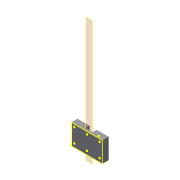
# Autodesk Inventor part: 04_Mount_Rail_Fastener
Saved by Autodesk Inventor 2019.4 (Build 234330000, 330)
## iProperties
Created: 2021-02-16
Part Number: 04_Mount_Rail_Fastener
Material: Generic
Document SubType Name: Modeling
Designer: diederichbenedict
Density: 1 g/cm^3
Appearance: Default
Author: diederichbenedict
Autodesk Inventor part; units mm, degrees
ref_plane "YZ Plane" through (0, 0, 0) normal (1, 0, 0) x (0, 1, 0)
ref_plane "XZ Plane" through (0, 0, 0) normal (0, 1, 0) x (-1, 0, 0)
ref_plane "Work Plane1" through (22.0339, 196.5, 8) normal (0, 0, 1) x (1, 0, 0)
sketch "Sketch1" plane through (22.0339, 196.5, 8) normal (0, 0, 1) x (1, 0, 0)
  circle A0 centre (5.4838, -190) radius 1.4 projected
  circle A1 centre (27.9838, -190) radius 1.4 projected
  circle A2 centre (-17.0162, -190) radius 1.4 projected
  line L0 (-22.0339, -196.5) -> (32.9661, -196.5) projected
  line L1 (32.9661, -196.5) -> (32.9661, -186.5) projected
  line L2 (-22.0339, -186.5) -> (32.9661, -186.5) projected
  line L3 (-22.0339, -196.5) -> (-22.0339, -186.5) projected
  circle A3 centre (27.9838, -165) radius 1.4 projected
  circle A4 centre (-17.0162, -165) radius 1.4 projected
  circle A5 centre (5.4838, -165) radius 1.4 projected
  line L4 (32.9661, -160.5) -> (32.9661, -169.5) projected
  line L5 (-22.0339, -160.5) -> (32.9661, -160.5) projected
  line L6 (-22.0339, -160.5) -> (-22.0339, -169.5) projected
  line L7 (32.9661, -169.5) -> (-22.0339, -169.5) projected
  line L8 (32.9661, -196.5) -> (-22.0339, -196.5)
  line L9 (-22.0339, -196.5) -> (-22.0339, -160.5)
  line L10 (-22.0339, -160.5) -> (32.9661, -160.5)
  line L11 (32.9661, -160.5) -> (32.9661, -196.5)
  constraints: 8 end point, 2 parallel, 1 horizontal, 1 perpendicular
extrude "Extrusion1" add sketch "Sketch1" along normal blind 4
sketch "Sketch2" plane through (22.0339, 196.5, 8) normal (0, 0, -1) x (-1, 0, 0)
  circle A0 centre (17.0162, -190) radius 1.4 projected
  circle A1 centre (-27.9838, -190) radius 1.4 projected
  circle A2 centre (-5.4838, -190) radius 1.4 projected
  circle A3 centre (-5.4838, -165) radius 1.4 projected
  circle A4 centre (17.0162, -165) radius 1.4 projected
  circle A5 centre (-27.9838, -165) radius 1.4 projected
  line L0 (-32.9661, -196.5) -> (-32.9661, -160.5) projected
  line L1 (22.0339, -196.5) -> (-32.9661, -196.5) projected
  line L2 (22.0339, -160.5) -> (22.0339, -196.5) projected
  line L3 (-32.9661, -160.5) -> (22.0339, -160.5) projected
  line L4 (22.0339, -196.5) -> (-32.9661, -196.5) projected
  line L5 (22.0339, -160.5) -> (0.6985, -160.5)
  line L6 (0.6985, -160.5) -> (0.6985, -196.5)
  line L7 (0.6985, -196.5) -> (22.0339, -196.5)
  line L8 (22.0339, -196.5) -> (22.0339, -160.5)
  line L9 (-32.9661, -196.5) -> (-32.9661, -160.5) projected
  line L10 (-32.9661, -160.5) -> (-11.6661, -160.5)
  line L11 (-11.6661, -160.5) -> (-11.6661, -196.5)
  line L12 (-11.6661, -196.5) -> (-32.9661, -196.5)
  line L13 (-32.9661, -196.5) -> (-32.9661, -160.5)
  line L14 (-11.4661, 0) -> (-11.4661, -200) projected
  line L15 (0.4985, 0) -> (0.4985, -200) projected
  dimension "d6" = 0.2
  dimension "d7" = 0.2
  constraints: 16 end point, 4 parallel, 2 horizontal, 2 perpendicular, 2 point on line
  measures "d6" distance between parallel lines of L15 L6
  measures "d7" distance between parallel lines of L14 L11
extrude "Extrusion2" add sketch "Sketch2" along normal blind 7 contours L0 L3 L11 L1 | L6 L3 L2 L1
sketch "Sketch3" plane through (22.0339, 196.5, 12) normal (0, 0, 1) x (1, 0, 0)
  circle A0 centre (-17.0162, -190) radius 1.4 projected
  circle A1 centre (27.9838, -190) radius 1.4 projected
  circle A2 centre (5.4838, -190) radius 1.4 projected
  circle A3 centre (5.4838, -165) radius 1.4 projected
  circle A4 centre (-17.0162, -165) radius 1.4 projected
  circle A5 centre (27.9838, -165) radius 1.4 projected
  line L0 (32.9661, -196.5) -> (32.9661, -160.5) projected
  line L1 (32.9661, -160.5) -> (-22.0339, -160.5) projected
  line L2 (-22.0339, -160.5) -> (-22.0339, -196.5) projected
  line L3 (-22.0339, -196.5) -> (32.9661, -196.5) projected
  circle A6 centre (28.987, -157.2) radius 1 projected
  circle A7 centre (28.987, -157.2) radius 1 projected
  circle A8 centre (50.837, -147.5) radius 1 projected
  line L4 (53.837, -158.2) -> (53.837, -154.2581) projected
  line L5 (53.837, -154.2581) -> (61.5817, -154.2581) projected
  line L6 (61.5817, -154.2581) -> (61.5817, -153.1829) projected
  line L7 (61.5817, -153.1829) -> (53.837, -153.1829) projected
  line L8 (53.837, -153.1829) -> (53.837, -149.448) projected
  line L9 (53.837, -149.448) -> (61.5817, -149.448) projected
  line L10 (61.5817, -149.448) -> (61.5817, -148.769) projected
  line L11 (61.5817, -148.769) -> (53.837, -148.769) projected
  line L12 (53.837, -148.769) -> (53.837, -146.5) projected
  arc A9 (53.837, -146.5) -> (51.837, -144.5) centre (51.837, -146.5) ccw projected
  line L13 (51.837, -144.5) -> (46.3523, -144.5) projected
  line L14 (46.3523, -144.5) -> (18.7709, -139.6366) projected
  line L15 (18.7709, -139.6366) -> (16.0392, -139.155) projected
  line L16 (16.0392, -139.155) -> (15.987, -139.4512) projected
  line L17 (15.987, -139.4512) -> (44.6201, -144.5) projected
  line L18 (44.6201, -144.5) -> (27.987, -144.5) projected
  arc A10 (27.987, -144.5) -> (25.987, -146.5) centre (27.987, -146.5) ccw projected
  line L19 (25.987, -146.5) -> (25.987, -158.2) projected
  arc A11 (25.987, -158.2) -> (27.987, -160.2) centre (27.987, -158.2) ccw projected
  line L20 (27.987, -160.2) -> (33.9661, -160.2) projected
  line L21 (33.9661, -164.2178) -> (33.9661, -160.2) projected
  line L22 (42.5677, -164.2178) -> (33.9661, -164.2178) projected
  line L23 (42.5677, -164.2178) -> (42.5677, -163.1992) projected
  line L24 (42.5677, -163.1992) -> (35.1545, -163.1992) projected
  line L25 (35.1545, -160.2) -> (35.1545, -163.1992) projected
  line L26 (35.1545, -160.2) -> (51.837, -160.2) projected
  arc A12 (51.837, -160.2) -> (53.837, -158.2) centre (51.837, -158.2) ccw projected
  line L27 (32.9661, -160.5) -> (-22.0339, -160.5) projected
  line L28 (20.9661, -160.5) -> (32.9661, -160.5)
  line L29 (32.9661, -160.5) -> (32.9661, -144.5)
  line L30 (32.9661, -144.5) -> (20.9661, -144.5)
  line L31 (20.9661, -144.5) -> (20.9661, -160.5)
  point P0 (-22.0339, -196.5)
  dimension "d8" = 12
  constraints: 8 end point, 3 point on line, 2 parallel, 1 horizontal, 1 perpendicular
  measures "d8" distance between parallel lines of L31 L29
ref_plane "Work Plane2" through (38.0184, 32.2776, 9) normal (0, 0, 1) x (1, 0, 0)
extrude "Extrusion3" add sketch "Sketch3" against normal up to surface (3 mm away) contours L1 L31 L30 A10 L19 A11 L20 L29 | L20 A11 L19 A10 L18 L29
sketch "Sketch4" plane through (55, 52, 9) normal (0, 0, -1) x (-1, 0, 0)
  circle A0 centre (3.9791, -12.7) radius 1 projected
  circle A1 centre (-17.8709, -3) radius 1 projected
  line L0 (-20.8709, -13.7) -> (-20.8709, -9.7581) projected
  line L1 (-20.8709, -9.7581) -> (-28.6156, -9.7581) projected
  line L2 (-28.6156, -9.7581) -> (-28.6156, -8.6829) projected
  line L3 (-28.6156, -8.6829) -> (-20.8709, -8.6829) projected
  line L4 (-20.8709, -8.6829) -> (-20.8709, -4.948) projected
  line L5 (-20.8709, -4.948) -> (-28.6156, -4.948) projected
  line L6 (-28.6156, -4.948) -> (-28.6156, -4.269) projected
  line L7 (-28.6156, -4.269) -> (-20.8709, -4.269) projected
  line L8 (-20.8709, -4.269) -> (-20.8709, -2) projected
  arc A2 (-18.8709, 0) -> (-20.8709, -2) centre (-18.8709, -2) ccw projected
  line L9 (-18.8709, 0) -> (-13.3862, 0) projected
  line L10 (-13.3862, 0) -> (14.1952, 4.8634) projected
  line L11 (14.1952, 4.8634) -> (16.9269, 5.345) projected
  line L12 (16.9269, 5.345) -> (16.9791, 5.0488) projected
  line L13 (16.9791, 5.0488) -> (-11.654, 0) projected
  line L14 (-11.654, 0) -> (4.9791, 0) projected
  arc A3 (6.9791, -2) -> (4.9791, 0) centre (4.9791, -2) ccw projected
  line L15 (6.9791, -2) -> (6.9791, -13.7) projected
  arc A4 (4.9791, -15.7) -> (6.9791, -13.7) centre (4.9791, -13.7) ccw projected
  line L16 (4.9791, -15.7) -> (-1, -15.7) projected
  line L17 (-1, -19.7178) -> (-1, -15.7) projected
  line L18 (-9.6016, -19.7178) -> (-1, -19.7178) projected
  line L19 (-9.6016, -19.7178) -> (-9.6016, -18.6992) projected
  line L20 (-9.6016, -18.6992) -> (-2.1884, -18.6992) projected
  line L21 (-2.1884, -15.7) -> (-2.1884, -18.6992) projected
  line L22 (-2.1884, -15.7) -> (-18.8709, -15.7) projected
  arc A5 (-20.8709, -13.7) -> (-18.8709, -15.7) centre (-18.8709, -13.7) ccw projected
  line L23 (12, -16) -> (55, -16) projected
  circle A6 centre (3.9791, -12.7) radius 1 projected
  circle A7 centre (49.9823, -45.5) radius 1.4 projected
  circle A8 centre (4.9823, -45.5) radius 1.4 projected
  circle A9 centre (27.4823, -45.5) radius 1.4 projected
  circle A10 centre (27.4823, -20.5) radius 1.4 projected
  circle A11 centre (49.9823, -20.5) radius 1.4 projected
  circle A12 centre (4.9823, -20.5) radius 1.4 projected
  line L24 (0, -52) -> (0, 0) projected
  line L25 (0, 0) -> (12, 0) projected
  line L26 (12, 0) -> (12, -16) projected
  line L27 (12, -16) -> (55, -16) projected
  line L28 (55, -16) -> (55, -52) projected
  line L29 (55, -52) -> (0, -52) projected
  line L30 (12, -16) -> (0, -16) projected
  line L31 (12, 0) -> (0, 0) projected
  line L32 (12, -16) -> (7.2, -16)
  line L33 (7.2, -16) -> (7.2, 0)
  line L34 (7.2, 0) -> (12, 0)
  line L35 (12, 0) -> (12, -16)
  point P0 (55, -52)
  dimension "d11" = 4.8
  constraints: 8 end point, 2 parallel, 1 horizontal, 1 perpendicular, 1 point on line
  measures "d11" distance of L33.end L34.end
extrude "Extrusion4" add sketch "Sketch4" along normal up to surface (8 mm away) contours L33 L25 L26 L30
body "Solid1"
